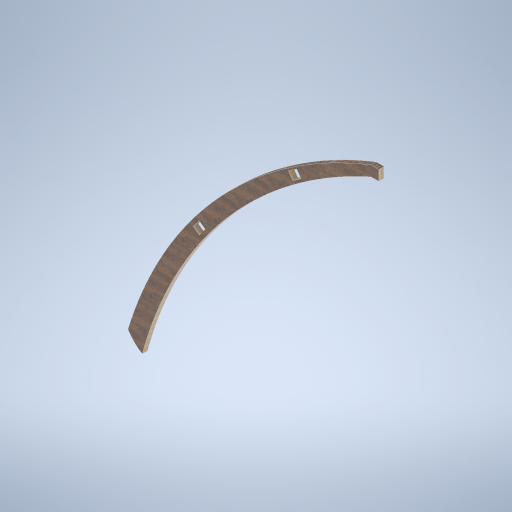
# Autodesk Inventor part: curve_beam_01
Saved by Autodesk Inventor 2024.2 (Build 282272000, 272)
## iProperties
Created: 2024-05-19
Part Number: curve_beam_01
Material: Wood (Maple)
Document SubType Name: Modeling
Designer: LOSTER_1
Density: 0.67 g/cm^3
Appearance: Natural Maple - Glossy Dark Tint
Author: LOSTER_1
Autodesk Inventor part; units mm, degrees
ref_plane "YZ Plane" through (0, 0, 0) normal (1, 0, 0) x (0, 1, 0)
ref_plane "XZ Plane" through (0, 0, 0) normal (0, 1, 0) x (-1, 0, 0)
ref_plane "XY Plane" through (0, 0, 0) normal (0, 0, 1) x (1, 0, 0)
sketch "Sketch1" plane through (0, 0, 0) normal (0, 0, 1) x (1, 0, 0)
  line L0 (4856.4349, 5392.3386) -> (4856.4349, 5192.3386)
  arc A0 (4706.4349, 5392.28) -> (-20.5961, 263.191) centre (7637.2096, -2051.5469) ccw
  ellipse E0 centre (665.286, 674.9746) end of major axis (665.286, -125.0254) minor radius 800 (-20.5961, 263.191) -> (256.6451, -12.7845) ccw
  arc A1 (4706.4349, 5192.3386) -> (256.6451, -12.7845) centre (7977.2775, -2108.4551) ccw
  line L1 (4706.4349, 5392.28) -> (4706.4349, 5392.3386)
  line L2 (4706.4349, 5392.3386) -> (4856.4349, 5392.3386)
  line L3 (4706.4349, 5192.3386) -> (4856.4349, 5192.3386)
  point P0 (0, 0)
  constraints: 8 end point, 4 point on circle, 2 centre point, 1 horizontal, 4 other
extrude "Extrusion1" add sketch "Sketch1" along normal blind 100
sketch "Sketch3" plane through (0, 0, 100) normal (0, 0, 1) x (1, 0, 0)
  point P0 (0, 0)
sketch "Sketch4" plane through (0, 0, 0) normal (0, 0, -1) x (-1, 0, 0)
  arc A0 (20.5961, 263.191) -> (-4706.4349, 5392.28) centre (-7637.2096, -2051.5469) ccw projected
  arc A1 (-256.6451, -12.7845) -> (-4706.4349, 5192.3386) centre (-7977.2775, -2108.4551) ccw projected
  ellipse E0 centre (-665.286, 674.9746) end of major axis (-665.286, -125.0254) minor radius 800 (-256.6451, -12.7845) -> (20.5961, 263.191) ccw projected
  line L0 (-3345.6941, 4477.7322) -> (-3181.8637, 4363.017)
  line L1 (-3181.8637, 4363.017) -> (-3095.8273, 4485.8898)
  line L2 (-3095.8273, 4485.8898) -> (-3259.6577, 4600.6051)
  line L3 (-3259.6577, 4600.6051) -> (-3345.6941, 4477.7322)
  line L4 (-3345.6941, 4477.7322) -> (-3095.8273, 4485.8898) construction
  line L5 (-3181.8637, 4363.017) -> (-3259.6577, 4600.6051) construction
  line L6 (-3345.6941, 4477.7322) -> (-3145.6941, 4477.7322) construction
  line L7 (-1357.1134, 2785.963) -> (-1242.3982, 2622.1326)
  line L8 (-1242.3982, 2622.1326) -> (-1365.271, 2536.0961)
  line L9 (-1365.271, 2536.0961) -> (-1479.9863, 2699.9265)
  line L10 (-1479.9863, 2699.9265) -> (-1357.1134, 2785.963)
  line L11 (-1357.1134, 2785.963) -> (-1365.271, 2536.0961) construction
  line L12 (-1242.3982, 2622.1326) -> (-1479.9863, 2699.9265) construction
  line L13 (-1357.1134, 2785.963) -> (-1157.1134, 2785.963) construction
  point P0 (0, 0)
  point P1 (-256.6451, -12.7845)
  point P2 (20.5961, 263.191)
  point P3 (-3220.7607, 4481.811)
  point P4 (-1361.1922, 2661.0296)
  dimension "d2" = 200
  dimension "d3" = 35
  dimension "d4" = 150
  dimension "d5" = 200
  dimension "d6" = 55
  dimension "d7" = 150
  constraints: 28 end point, 4 midpoint, 4 parallel, 2 coincident, 2 equal length, 2 horizontal, 2 perpendicular, 1 other
  measures "d2" distance of L0.start L0.end
  measures "d3" angle of L0 L6
  measures "d4" distance of L1.end L0.end
  measures "d5" distance of L7.start L7.end
  measures "d6" angle of L7 L13
  measures "d7" distance of L7.end L8.end
extrude "Extrusion2" cut sketch "Sketch4" against normal through all
body "Solid1"
